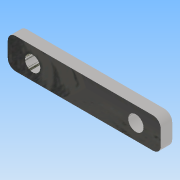
# Autodesk Inventor part: cell
Saved by Autodesk Inventor 2015 (Build 190159000, 159)
## iProperties
Created: 2017-02-14
Part Number: cell
Material: Générique
Document SubType Name: Modeling
Designer: Gregwar
Density: 1 g/cm^3
Appearance: Par défaut
Author: Gregwar
Autodesk Inventor part; units mm, degrees
ref_plane "YZ Plane" through (0, 0, 0) normal (1, 0, 0) x (0, 1, 0)
ref_plane "XZ Plane" through (0, 0, 0) normal (0, 1, 0) x (-1, 0, 0)
ref_plane "XY Plane" through (0, 0, 0) normal (0, 0, 1) x (1, 0, 0)
sketch "Esquisse1" plane through (0, 0, 0) normal (0, 1, 0) x (-1, 0, 0)
  line L0 (0, 0) -> (40, 0)
  line L1 (40, 0) -> (40, -8)
  line L2 (40, -8) -> (0, -8)
  line L3 (0, -8) -> (0, 0)
  line L4 (40, -4) -> (0, -4) construction
  line L5 (20, 0) -> (20, -8) construction
  circle A0 centre (33.5, -4) radius 2
  circle A1 centre (6.5, -4) radius 2
  dimension "d0" = 8
  dimension "d1" = 40
  dimension "d2" = 27
  dimension "d3" = 4
  constraints: 12 end point, 4 midpoint, 2 centre point, 2 parallel, 1 horizontal, 1 perpendicular, 1 point on line, 1 symmetric about line, 1 other
  measures "d0" distance of L2.end L0.start
  measures "d1" distance of L0.start L0.end
  measures "d2" distance of A1.centre A0.centre
  measures "d3" diameter of A0
extrude "Extrusion1" add sketch "Esquisse1" along normal blind 3
fillet "Congé1" radius 2 4 edges at (0, 1.5, 0) (0, 1.5, -8) (-40, 1.5, -8) (-40, 1.5, 0)
